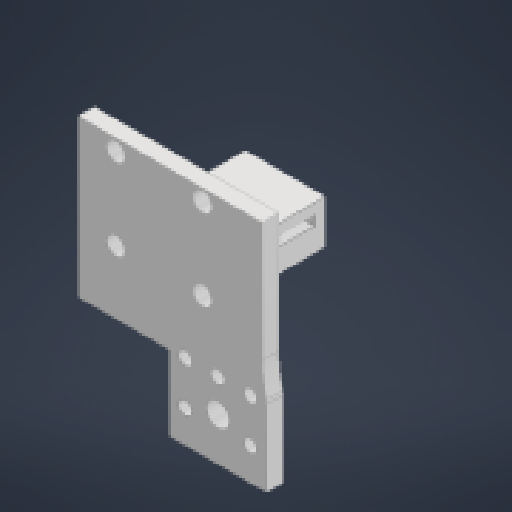
# Autodesk Inventor part: top plate normal
Saved by Autodesk Inventor 2024 (Build 280153000, 153)
## iProperties
Created: 2024-06-01
Part Number: top plate normal
Material: Generic
Document SubType Name: Modeling
Designer: mateu
Density: 1 g/cm^3
Appearance: Default
Author: mateu
Autodesk Inventor part; units mm, degrees
ref_plane "YZ Plane" through (0, 0, 0) normal (1, 0, 0) x (0, 1, 0)
ref_plane "XZ Plane" through (0, 0, 0) normal (0, 1, 0) x (-1, 0, 0)
ref_plane "XY Plane" through (0, 0, 0) normal (0, 0, 1) x (1, 0, 0)
sketch "Sketch1" plane through (0, 0, 0) normal (0, 0, 1) x (1, 0, 0)
  line L0 (-2.875, 15.3) -> (-2.875, 20.2) projected
  line L1 (-2.875, 15.3) -> (27.025, 15.3) projected
  line L2 (27.025, 15.3) -> (27.025, 20.2) projected
  line L3 (-2.875, 20.2) -> (27.025, 20.2) projected
  circle A0 centre (4.075, 17.5) radius 1.75 projected
  circle A1 centre (20.075, 17.5) radius 1.75 projected
  line L4 (-2.875, 29.8) -> (-2.875, 34.7) projected
  line L5 (-2.875, 29.8) -> (27.025, 29.8) projected
  line L6 (27.025, 29.8) -> (27.025, 34.7) projected
  line L7 (-2.875, 34.7) -> (27.025, 34.7) projected
  circle A2 centre (20.075, 32.5) radius 1.75 projected
  circle A3 centre (4.075, 32.5) radius 1.75 projected
  line L8 (-6.875, 34.7) -> (27.025, 34.7)
  line L9 (27.025, 29.8) -> (27.025, 20.2)
  line L10 (27.025, 15.3) -> (10.325, 15.3)
  line L11 (10.325, 15.3) -> (10.325, 14.3)
  line L12 (10.325, 14.3) -> (27.025, 14.3)
  line L13 (27.025, 14.3) -> (27.025, 15.3)
  line L14 (-6.875, 34.7) -> (-6.875, 12.6453)
  line L15 (-6.875, 34.7) -> (20.1667, 34.7) construction
  arc A4 (-7.3214, 7.9419) -> (-6.875, 12.6453) centre (-31.875, 12.6453) ccw
  arc A5 (-6.875, 12.6453) -> (-7.5893, 6.712) centre (-31.875, 12.6453) ccw construction
  line L16 (-6.875, 12.6453) -> (-6.875, 7.6583) construction
  line L17 (10.325, 6) -> (10.325, 14.3)
  line L18 (-2.875, 15) -> (27.025, 15) projected
  line L19 (-2.875, 14.8) -> (27.025, 14.8)
  line L20 (10.325, 6) -> (10.325, -6)
  line L21 (-7.675, 7.05) -> (-7.675, -8.5199)
  line L22 (-6.2394, 1.4274) -> (-6.2394, -1.4274)
  arc A6 (-6.2394, 1.4274) -> (-7.1366, 4.2853) centre (-11.2394, 1.4274) ccw
  arc A7 (-4.675, 9) -> (-7.1366, 4.2853) centre (-4.675, 6) ccw
  line L23 (7.325, 9) -> (-4.675, 9)
  arc A8 (9.8134, 4.3243) -> (7.325, 9) centre (7.325, 6) ccw
  arc A9 (9.8134, 4.3243) -> (8.9606, 1.5314) centre (13.9606, 1.5314) ccw
  line L24 (8.9606, -1.5314) -> (8.9606, 1.5314)
  arc A10 (8.9606, -1.5314) -> (9.8134, -4.3243) centre (13.9606, -1.5314) ccw
  line L25 (10.325, -6) -> (10.325, -8.01)
  arc A11 (10.325, -6) -> (9.8134, -4.3243) centre (7.325, -6) ccw
  line L26 (10.325, -8.01) -> (-7.675, -8.01)
  line L27 (-7.675, -6) -> (-7.675, -8.01)
  arc A12 (-7.1366, -4.2853) -> (-7.675, -6) centre (-4.675, -6) ccw
  arc A13 (-7.1366, -4.2853) -> (-6.2394, -1.4274) centre (-11.2394, -1.4274) ccw
  arc A14 (-7.5893, 6.712) -> (-7.3214, 7.9419) centre (-31.875, 12.6453) ccw
  circle A15 centre (7.325, 5.9594) radius 1
  circle A16 centre (1.325, 5.9594) radius 1.05
  circle A17 centre (-4.675, 5.9594) radius 0.85
  circle A18 centre (-4.675, -2.0406) radius 0.85
  circle A19 centre (1.325, -0.0406) radius 2.1
  circle A20 centre (7.325, -2.0406) radius 0.85
  circle A21 centre (-4.675, 6) radius 1.15 projected
  circle A22 centre (1.325, -0.0406) radius 3.1 projected
  arc A23 (-2.5188, 3.9142) -> (-3.925, 0.4379) centre (1.075, 0.4379) ccw projected
  arc A24 (-2.5188, 3.9142) -> (-4.675, 9) centre (-4.675, 6) ccw projected
  line L28 (7.325, 9) -> (-4.675, 9) projected
  arc A25 (7.325, 9) -> (5.1687, 3.9142) centre (7.325, 6) ccw projected
  arc A26 (6.575, 0.4379) -> (5.1687, 3.9142) centre (1.575, 0.4379) ccw projected
  line L29 (6.575, 0.4379) -> (6.575, -0.7085) projected
  arc A27 (5.325, -4.0157) -> (6.575, -0.7085) centre (1.575, -0.7085) ccw projected
  arc A28 (5.325, -4.0157) -> (4.9856, -7.515) centre (7.575, -6) ccw projected
  arc A29 (4.9856, -7.515) -> (5.8488, -8.01) centre (5.8488, -7.01) ccw projected
  line L30 (-3.1988, -8.01) -> (5.8488, -8.01) projected
  arc A30 (-3.1988, -8.01) -> (-2.3356, -7.515) centre (-3.1988, -7.01) ccw projected
  arc A31 (-2.3356, -7.515) -> (-2.675, -4.0157) centre (-4.925, -6) ccw projected
  arc A32 (-3.925, -0.7085) -> (-2.675, -4.0157) centre (1.075, -0.7085) ccw projected
  line L31 (-3.925, -0.7085) -> (-3.925, 0.4379) projected
  circle A33 centre (7.325, 6) radius 1.15 projected
  arc A34 (4.9856, -7.515) -> (5.8488, -8.01) centre (5.8488, -7.01) ccw projected
  arc A35 (5.325, -4.0157) -> (4.9856, -7.515) centre (7.575, -6) ccw projected
  arc A36 (5.325, -4.0157) -> (6.575, -0.7085) centre (1.575, -0.7085) ccw projected
  line L32 (6.575, -0.7085) -> (6.575, 0.4379) projected
  arc A37 (6.575, 0.4379) -> (5.1687, 3.9142) centre (1.575, 0.4379) ccw projected
  arc A38 (9.8, 4.3046) -> (5.1687, 3.9142) centre (7.325, 6) ccw projected
  arc A39 (9.8, 4.3046) -> (8.925, 1.4789) centre (13.925, 1.4789) ccw projected
  line L33 (8.925, 1.4789) -> (8.925, -1.4789) projected
  arc A40 (8.925, -1.4789) -> (9.8, -4.3046) centre (13.925, -1.4789) ccw projected
  arc A41 (10.325, -6) -> (9.8, -4.3046) centre (7.325, -6) ccw projected
  line L34 (10.325, -6) -> (10.325, -8.01) projected
  line L35 (10.325, -8.01) -> (5.8488, -8.01) projected
  circle A42 centre (7.325, -0.0515) radius 0.4 projected
  circle A43 centre (7.325, 6) radius 1.25 projected
  circle A44 centre (7.325, -6) radius 1.25 projected
  circle A45 centre (7.325, -2.0406) radius 0.85 projected
  circle A46 centre (-4.675, -2.0406) radius 0.85 projected
  point P0 (10.135, 15.3)
  point P1 (10.325, 15.3)
  point P2 (10.325, 14.8)
  point P3 (-7.675, 6)
  dimension "d16" = 1
  dimension "d22" = 90
  dimension "d23" = 50
  dimension "d24" = 0.2
  constraints: 38 end point, 23 point on circle, 17 centre point, 5 tangent, 5 vertical, 4 horizontal, 3 parallel, 2 collinear, 2 perpendicular, 2 point on line, 42 other
  measures "d16" distance of L11.end L10.end
  measures "d22" angle of L14 L15
  measures "d23" diameter of A4
  measures "d24" distance between parallel lines of L18 L19
extrude "Extrusion1" add sketch "Sketch1" along normal blind 3 contours L1 L11 L17 A8 L23 A7 A14 A4 L14 L8 L4 L5 L9 L3 L0 | L0 L3 L2 L1 | L1 L13 L18 L11 | L18 L13 L19 L11 | L5 L4 L7 L6 | L20 A11 A10 L24 A9 A8 | A8 A9 A39 L33 A40 A10 A11 L25 L26 A29 A28 A27 L29 A26 A25 | A25 A26 L29 A27 A28 A29 L26 A30 A31 A32 L31 A23 A24 L23 | A9 L24 A10 A40 L33 A39 | A24 A23 L31 A32 A31 A30 L26 L21 A12 A13 L22 A6 A7 | A7 A6 L22 A13 A12 L21 | A0 | A1 | A2 | A3 | A15 | A16 | A17 | A18 | A20 | A21 | A22 | A33 | A42 | A43 | A44
sketch "Sketch6" plane through (27.025, 14.8, 0) normal (1, 0, 0) x (0, 0, -1)
  line L0 (0, 0) -> (-3, 0) projected
  line L1 (-3, 0) -> (7.7, 0)
  line L2 (7.7, 0) -> (7.7, -1)
  line L3 (7.7, -1) -> (27.831, -1)
  line L4 (21.831, -2.2) -> (21.831, -2.2)
  line L5 (10.331, -3.1) -> (10.331, -3.8184)
  line L6 (17.931, -3.1) -> (17.931, -3.8184)
  line L7 (10.331, -2.2) -> (17.931, -2.2)
  line L8 (17.931, -2.2) -> (17.931, -5.7)
  line L9 (17.931, -5.7) -> (10.331, -5.7)
  line L10 (10.331, -5.7) -> (10.331, -2.2)
  line L11 (27.831, -1) -> (27.831, -9)
  line L12 (27.831, -9) -> (0, -9)
  line L13 (0, -9) -> (0, 0)
  line L14 (7.7, 0) -> (0, 0)
  line L15 (0, -9) -> (-3, -9)
  line L16 (-3, -9) -> (-3, 0)
  line L17 (0, 0) -> (-3, 0)
  line L18 (19.431, -2.9) -> (25.831, -2.9)
  line L19 (25.831, -2.9) -> (25.831, -4.7)
  line L20 (25.831, -4.7) -> (19.431, -4.7)
  line L21 (19.431, -4.7) -> (19.431, -2.9)
  line L22 (11.131, -3.1) -> (11.131, -3.8184) projected
  line L23 (11.131, -3.8184) -> (17.131, -3.8184) projected
  line L24 (17.131, -3.1) -> (17.131, -3.8184) projected
  line L25 (11.131, -3.1) -> (17.131, -3.1) projected
  line L26 (19.631, -3.1) -> (19.631, -3.8184) projected
  line L27 (19.631, -3.1) -> (25.631, -3.1) projected
  point P0 (0, -14.8)
  point P1 (7.7, 0.2)
  dimension "d25" = 1
  dimension "d36" = 8
  dimension "d54" = 1.8
  dimension "d59" = 7.6
  dimension "d60" = 0.8
  dimension "d61" = 6.4
  dimension "d62" = 0.2
  dimension "d63" = 0.2
  dimension "d88" = 2
  constraints: 42 end point, 6 perpendicular, 4 collinear, 4 horizontal, 4 parallel, 1 coincident, 1 point on line, 1 vertical, 1 vertical alignment, 1 other
  measures "d25" distance of L2.start L2.end
  measures "d36" distance of L3.end L11.end
  measures "d54" distance between parallel lines of L20 L18
  measures "d59" distance between parallel lines of L8 L10
  measures "d60" distance between parallel lines of L5 L22
  measures "d61" distance between parallel lines of L21 L19
  measures "d62" distance between parallel lines of L21 L26
  measures "d63" distance between parallel lines of L18 L27
  measures "d88" distance between parallel lines of L11 L19
extrude "Extrusion2" add sketch "Sketch6" against normal blind 14.7 contours L13 L15 L16 L0 | L1 L2 L3 L11 L12 L13
sketch "Sketch12" plane through (0, 0, 3) normal (0, 0, 1) x (1, 0, 0)
  arc A0 (23.1194, 9.1) -> (21.3306, 9.1) centre (22.225, 9.2) ccw
  line L0 (27.025, 9.1) -> (23.1194, 9.1)
  line L1 (27.025, 12.6) -> (27.025, 9.1)
  line L2 (27.025, 12.6) -> (12.625, 12.6)
  line L3 (12.625, 9.1) -> (12.625, 12.6)
  line L4 (16.5306, 9.1) -> (12.625, 9.1)
  arc A1 (18.3194, 9.1) -> (16.5306, 9.1) centre (17.425, 9.2) ccw
  line L5 (21.3306, 9.1) -> (18.3194, 9.1)
  circle A2 centre (24.525, 8.3) radius 1
  circle A3 centre (15.125, 8.3) radius 1
  line L6 (27.025, 34.7) -> (27.025, 5.8)
  line L7 (27.025, 5.8) -> (12.325, 5.8) projected
  point P0 (0, 0)
  point P1 (10.625, 5.8)
  point P2 (10.325, 5.8)
  dimension "d72" = 2
  dimension "d73" = 2
  dimension "d74" = 2.5
  dimension "d75" = 2.5
  dimension "d83" = 2.5
  constraints: 14 end point, 5 centre point, 4 point on circle, 1 horizontal alignment
  measures "d72" diameter of A2
  measures "d73" diameter of A3
  measures "d74" distance from line of L6 A2.centre
  measures "d75" distance from line of L3 A3.centre
  measures "d83" distance from line of L7 A2.centre
hole "Hole3" at (24.525, 8.3, 3) at (15.125, 8.3, 3) direction (0, 0, -1) diameter 2.2 depth 40 countersink diameter 4.4 countersink angle 90 clearance for "Countersunk Flat Head Screw ISO 2009/7046" size "M2" standard "ISO"
sketch "Sketch13" plane through (27.025, 10.1, -19.431) normal (0, 0, -1) x (-1, 0, 0)
  circle A0 centre (2.5, -1.8) radius 1.1 projected
  circle A1 centre (11.9, -1.8) radius 1.1 projected
  line L0 (0, -4.3) -> (14.7, -4.3) projected
  line L1 (5.55, -8.6) -> (5.55, 0)
  line L2 (5.55, 0) -> (9.15, 0)
  line L3 (9.15, 0) -> (9.15, -8.6)
  line L4 (9.15, -8.6) -> (5.55, -8.6)
  line L5 (5.55, -8.6) -> (9.15, 0) construction
  line L6 (5.55, 0) -> (9.15, -8.6) construction
  circle A2 centre (3.75, -1.8) radius 1.8
  circle A3 centre (10.95, -1.8) radius 1.8
  circle A4 centre (11.9, -1.8) radius 1.1 projected
  circle A5 centre (2.5, -1.8) radius 1.1 projected
  line L7 (14.7, 3.7) -> (14.7, -4.3) projected
  line L8 (0, 3.7) -> (14.7, 3.7) projected
  line L9 (0, -4.3) -> (0, 3.7) projected
  line L10 (0, -4.3) -> (14.7, -4.3) projected
  line L11 (0, 0) -> (14.7, 0) projected
  circle A6 centre (10.95, -1.8) radius 3.6
  line L12 (0, 1.8) -> (14.7, 1.8) projected
  circle A7 centre (3.75, -1.8) radius 3.6
  circle A8 centre (3.75, -1.8) radius 3.8
  circle A9 centre (10.95, -1.8) radius 3.8
  circle A10 centre (7.35, 1.3749) radius 1
  point P0 (27.025, -10.1)
  point P1 (7.35, -4.3)
  point P2 (16.7, -4.3)
  point P3 (16.7, 0)
  point P4 (3.75, 0)
  point P5 (5.55, -1.8)
  point P6 (5.55, -4.3)
  point P7 (9.15, -4.3)
  point P8 (9.15, -1.8)
  point P9 (10.95, 0)
  point P10 (16.7, 1.8)
  point P11 (4.9666, 1.8)
  point P12 (6.6, 0.7135)
  point P13 (8.1, 0.7135)
  point P14 (9.7334, 1.8)
  dimension "d84" = 3.6
  dimension "d85" = 3.6
  dimension "d89" = 0.2
  dimension "d90" = 0.2
  dimension "d91" = 2
  constraints: 12 end point, 7 centre point, 6 tangent, 3 midpoint, 2 coincident, 2 horizontal alignment, 2 parallel, 1 equal radius, 1 perpendicular, 1 other
  measures "d84" distance of L1.end L2.end
  measures "d85" diameter of A2
  measures "d89" radial gap between concentric circles of A7 A8
  measures "d90" radial gap between concentric circles of A6 A9
  measures "d91" diameter of A10
extrude "Extrusion5" cut sketch "Sketch13" along normal blind 6.4 contours L11 L1 A2 | L1 L2 A7 A9 L0 | L2 A8 A9 A7 | A7 A9 A8 L0 | L2 A9 A8 | A9 A8 A6 A7 | A7 A9 | A8 A9 L0 | A7 A6 A8 A9 | L2 A6 A8 A9 | A6 A8 | A9 A8 A6 L0 | L2 L3 L0 A6 A8 | L11 A3 L3
extrude "Extrusion6" add sketch "Sketch13" along normal blind 6.4 contours L12 A10 A8 | L12 A10 | L12 A9 A10 picked at (7.3097, 1.3274)
sketch "Sketch15" plane through (27.025, 10.1, -19.431) normal (0, 0, -1) x (-1, 0, 0)
  arc A0 (9.7334, 1.8) -> (8.1, 0.7135) centre (10.95, -1.8) ccw projected
  arc A1 (6.6, 0.7135) -> (8.1, 0.7135) centre (7.35, 1.3749) ccw projected
  arc A2 (6.6, 0.7135) -> (4.9666, 1.8) centre (3.75, -1.8) ccw projected
  line L0 (0, 1.8) -> (4.9666, 1.8) projected
  line L1 (0, 0) -> (0, 1.8) projected
  line L2 (0, 0) -> (3.75, 0) projected
  arc A3 (5.55, -1.8) -> (3.75, 0) centre (3.75, -1.8) ccw projected
  line L3 (5.55, -1.8) -> (5.55, -4.3) projected
  line L4 (9.15, -4.3) -> (5.55, -4.3) projected
  line L5 (9.15, -4.3) -> (9.15, -1.8) projected
  arc A4 (10.95, 0) -> (9.15, -1.8) centre (10.95, -1.8) ccw projected
  line L6 (10.95, 0) -> (14.7, 0) projected
  line L7 (14.7, 1.8) -> (14.7, 0) projected
  line L8 (9.7334, 1.8) -> (14.7, 1.8) projected
  line L9 (9.1539, -2.5987) -> (9.1539, -3.389)
  line L10 (9.1539, -3.389) -> (9.1539, -2.5987)
  line L11 (9.4125, -3.4593) -> (9.1539, -3.389)
  arc A5 (9.409, -4.5313) -> (9.4125, -3.4593) centre (9.2668, -3.9949) ccw
  arc A6 (9.409, -4.5313) -> (9.4125, -3.4593) centre (9.2668, -3.9949) ccw
  line L12 (9.409, -4.5313) -> (9.15, -4.6)
  arc A7 (9.409, -4.5313) -> (9.4125, -3.4593) centre (9.2668, -3.9949) ccw
  line L13 (9.2668, -3.9949) -> (9.409, -4.5313) construction
  line L14 (9.2668, -3.9949) -> (9.4125, -3.4593) construction
  line L15 (0, 24.6) -> (33.9, 24.6) projected
  line L16 (9.4125, -1.4593) -> (9.1539, -1.389)
  arc A8 (9.409, -2.5313) -> (9.4125, -1.4593) centre (9.2668, -1.9949) ccw
  line L17 (9.409, -2.5313) -> (9.15, -2.6)
  arc A9 (9.5346, -0.688) -> (9.195, -1.4002) centre (10.95, -1.8) ccw
  arc A10 (9.5898, -0.7708) -> (10.5422, -0.2789) centre (10, -0.397) ccw
  line L18 (10.5422, -0.2789) -> (10.4852, -0.017)
  line L19 (9.5898, -0.7708) -> (9.4092, -0.5728)
  line L20 (7.35, 0.3749) -> (7.35, -4.3)
  line L21 (5.2875, -3.4593) -> (5.5461, -3.389)
  arc A11 (5.2875, -3.4593) -> (5.291, -4.5313) centre (5.4332, -3.9949) ccw
  line L22 (5.2875, -1.4593) -> (5.5461, -1.389)
  arc A12 (5.2875, -1.4593) -> (5.291, -2.5313) centre (5.4332, -1.9949) ccw
  line L23 (5.291, -2.5313) -> (5.55, -2.6)
  arc A13 (4.1578, -0.2789) -> (5.1102, -0.7708) centre (4.7, -0.397) ccw
  line L24 (4.1578, -0.2789) -> (4.2148, -0.017)
  line L25 (5.1102, -0.7708) -> (5.2908, -0.5728)
  line L26 (5.5461, -3.389) -> (5.5695, -3.3826)
  line L27 (9.1539, -3.389) -> (9.1416, -3.3857)
  line L28 (10.7656, -0.0095) -> (10.5114, -0.6126)
  line L29 (2.891, -0.2182) -> (4.1578, -0.5151)
  line L30 (33.9, 24.6) -> (33.9, 2.5453) projected
  arc A14 (33.9, 2.5453) -> (34.6143, -3.388) centre (58.9, 2.5453) ccw projected
  arc A15 (34.7, -4.1) -> (34.6143, -3.388) centre (31.7, -4.1) ccw projected
  line L31 (34.7, -4.1) -> (34.7, -18.11) projected
  line L32 (34.7, -18.11) -> (16.7, -18.11) projected
  line L33 (16.7, -18.11) -> (16.7, 4.7) projected
  line L34 (0, 24.6) -> (0, -4.3) projected
  line L35 (0, -4.3) -> (14.7, -4.3) projected
  line L36 (16.7, 4.7) -> (14.7, 4.7) projected
  line L37 (14.7, -4.3) -> (14.7, 4.7) projected
  point P0 (27.025, -10.1)
  point P1 (10.4943, -0.0586)
  point P2 (9.5252, -0.7)
  point P3 (10.4943, -0.0586)
  point P4 (9.15, -2.6)
  point P5 (9.15, -3.3879)
  point P6 (4.2057, -0.0586)
  point P7 (5.1748, -0.7)
  point P8 (5.55, -2.6)
  point P9 (5.505, -1.4002)
  point P10 (5.55, -3.3879)
  point P11 (4.9696, -4.3)
  point P12 (5.55, -4.3)
  point P13 (9.15, -4.3)
  point P14 (9.7304, -4.3)
  dimension "d95" = 0.555
  dimension "d98" = 105.21
  dimension "d101" = 30.056
  dimension "d103" = 0.7903
  dimension "d105" = 149.944
  dimension "d106" = 0.2586
  dimension "d107" = 0.113
  dimension "d109" = 0.3
  dimension "d112" = 2
  dimension "d117" = 0.789
  dimension "d120" = 62.5
  constraints: 40 end point, 25 point on circle, 14 symmetric about line, 9 centre point, 3 coincident, 3 point on line, 3 tangent, 1 concentric, 1 equal length, 1 perpendicular, 1 vertical, 21 other
  measures "d95" radius of A6
  measures "d98" angle of L9 L11
  measures "d101" angle of L12 L11
  measures "d103" distance of L9.start L9.end
  measures "d105" angle of L13 L14
  measures "d106" horizontal distance of L11.start L9.end
  measures "d107" distance from line of L9 A5.centre
  measures "d109" distance of L12.end L4.start
  measures "d112" distance of L11.start L16.start
  measures "d117" distance of A9.end A9.start
extrude "Extrusion7" cut sketch "Sketch15" along normal blind 6.4 contours L5 L27 L11 A5 L35 | L35 A11 L21 L26 L3 | L28 A10 L18 A4 | L18 A10 L19 A4 | L5 A4 L16 A8 L17 | L23 A12 L22 A3 L3 | A3 L25 A13 L24
fillet "Fillet1" radius 0.2 6 edges at (21.475, 7.5, -22.631) (21.52, 8.6998, -22.631) (21.8502, 9.4, -22.631) (17.875, 7.5, -22.631) (17.83, 8.6998, -22.631) (17.4998, 9.4, -22.631)
extrude "Extrusion8" add sketch "Sketch6" against normal up to surface (16.7 mm away) contours L13 L15 L16 L0
sketch "Sketch16" plane through (0, 0, 0) normal (0, 0, -1) x (-1, 0, 0)
  circle A0 centre (4.675, -2.0406) radius 1.05 projected
  circle A1 centre (-7.325, -2.0406) radius 1.05 projected
  circle A2 centre (-7.325, 5.9594) radius 1.05 projected
  circle A3 centre (4.675, 5.9594) radius 1.05 projected
  circle A4 centre (-1.325, -0.0406) radius 2.1 projected
  circle A5 centre (-1.325, 5.9594) radius 1.05 projected
  circle A6 centre (4.675, -2.0406) radius 1.05 projected
  arc A7 (-9.8, -4.3046) -> (-10.325, -6) centre (-7.325, -6) ccw projected
  arc A8 (-9.8, -4.3046) -> (-8.925, -1.4789) centre (-13.925, -1.4789) ccw projected
  line L0 (-8.925, -1.4789) -> (-8.925, 1.4789) projected
  arc A9 (-8.925, 1.4789) -> (-9.8, 4.3046) centre (-13.925, 1.4789) ccw projected
  line L1 (-7.325, 9) -> (4.675, 9) projected
  arc A10 (7.15, 4.3046) -> (6.275, 1.4789) centre (11.275, 1.4789) ccw projected
  line L2 (6.275, 1.4789) -> (6.275, -1.4789) projected
  arc A11 (6.275, -1.4789) -> (7.15, -4.3046) centre (11.275, -1.4789) ccw projected
  arc A12 (7.675, -6) -> (7.15, -4.3046) centre (4.675, -6) ccw projected
  line L3 (7.675, -6) -> (7.675, -8.01) projected
  line L4 (-10.325, -8.01) -> (7.675, -8.01) projected
  line L5 (-10.325, -6) -> (-10.325, -8.01) projected
  point P0 (0, 0)
hole "Hole4" at (-4.675, -2.0406, 0) at (7.325, -2.0406, 0) at (7.325, 5.9594, 0) at (1.325, 5.9594, 0) at (-4.675, 5.9594, 0) direction (0, 0, 1) diameter 2.4 depth 3.5 tip angle 118 clearance for "Countersunk Flat Head Screw ISO 2009/7046" size "M2" standard "ISO"
sketch "Sketch17" plane through (0, 0, 3) normal (0, 0, -1) x (-1, 0, 0)
  circle A0 centre (-4.075, 17.5) radius 1.25 projected
  circle A1 centre (-20.075, 17.5) radius 1.25 projected
  circle A2 centre (-20.075, 32.5) radius 1.25 projected
  circle A3 centre (-4.075, 32.5) radius 1.25 projected
  point P0 (0, 0)
hole "Hole5" at (4.075, 32.5, 3) at (20.075, 32.5, 3) at (20.075, 17.5, 3) at (4.075, 17.5, 3) direction (0, 0, -1) diameter 3.4 depth 3.5 tip angle 118 clearance for "Countersunk Flat Head Screw ISO 2009/7046" size "M3" standard "ISO"
mirror "Mirror1" about plane through (0, 0, 0) normal (1, 0, 0) remove original yes
body "Solid1"
